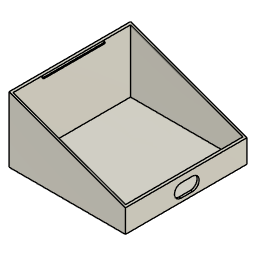
xbox-elite-s2-controller-holder v1 (Autodesk Fusion 360 design; units mm, degrees)
Autodesk Fusion 360 part; units mm, degrees
sketch "Sketch1" plane through (0, 0, 0) normal (0, 0, 1) x (1, 0, 0)
  line L0 (-95, 25) -> (-38, 25)
  line L1 (-38, 25) -> (-38, 84.5)
  line L2 (-38, 84.5) -> (-95, 84.5)
  line L3 (-95, 84.5) -> (-95, 25)
  dimension "d1" = 57
  dimension "d2" = 59.5
  constraint horizontal L0
  constraint vertical L1
  constraint horizontal L2
  constraint vertical L3
  measures "d1" distance of L0.start L0.end
  measures "d2" distance of L0.start L2.end
extrude "Extrude1" add sketch "Sketch1" along normal blind 32
shell "Shell1" thickness 1 removed faces 1 at (-76, 64.6667, 32)
draft "Draft1" angle -20 neutral plane through (-95, 84.5, 0) pull (-1, 0, 0) 1 faces at (-94.6667, 64.3333, 32)
sketch "Sketch2" plane through (-38, 0, 0) normal (1, 0, 0) x (0, 1, 0)
  line L0 (25, 0) -> (84.5, 0)
  line L1 (84.5, 0) -> (84.5, 11.2537)
  line L2 (84.5, 11.2537) -> (25, 11.2537)
  line L3 (25, 11.2537) -> (25, 0)
  line L4 (52.25, 1.75) -> (57.85, 1.75)
  arc A0 (57.85, 1.75) -> (57.85, 8.25) centre (57.85, 5) ccw
  line L5 (57.85, 8.25) -> (52.25, 8.25)
  arc A1 (52.25, 8.25) -> (52.25, 1.75) centre (52.25, 5) ccw
  line L6 (49, 5) -> (61.1, 5) construction
  dimension "d8" = 6.5
  constraint tangent L4 A0
  constraint tangent A0 L5
  constraint parallel L4 L5
  constraint tangent L5 A1
  constraint tangent L4 A1
  constraint midpoint A1 L6.start
  constraint midpoint A0 L6.end
  constraint parallel L2 L6
  measures "d8" diameter of A0
extrude "Extrude2" cut sketch "Sketch2" against normal blind 1 contours L4 A0 L5 A1
sketch "Sketch3" plane through (-94, 0, 0) normal (1, 0, 0) x (0, 1, 0)
  line L0 (26, 1) -> (83.5, 1)
  line L1 (83.5, 1) -> (83.5, 31.636)
  line L2 (83.5, 31.636) -> (26, 31.636)
  line L3 (26, 31.636) -> (26, 1)
  line L4 (40, 31) -> (70.0439, 31)
  line L5 (70.0439, 31) -> (70.0439, 31.636)
  line L6 (70.0439, 31.636) -> (40, 31.636)
  line L7 (40, 31.636) -> (40, 31)
  dimension "d13" = 0.636
  dimension "d14" = 30.0439
  constraint horizontal L4
  constraint vertical L5
  constraint horizontal L6
  constraint vertical L7
  constraint coincident L2 L5.end
  measures "d13" distance of L4.start L6.end
  measures "d14" distance of L4.start L4.end
extrude "Extrude3" add sketch "Sketch3" along normal blind 1 contours L2 L4 L5 L6 L7
